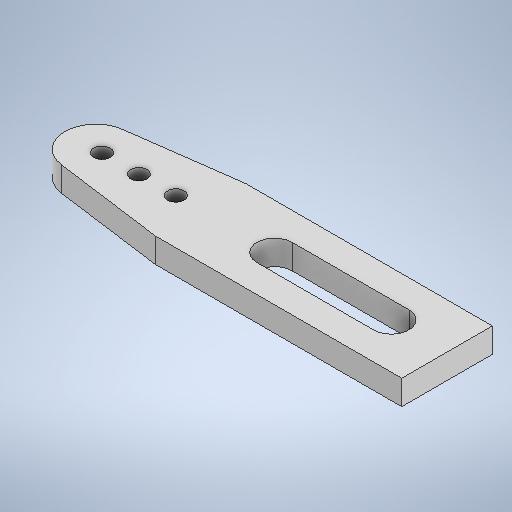
# Autodesk Inventor part: MMAE 232 Assignment 2_Servo Horn 1 - Dylan Tamras
Saved by Autodesk Inventor 2025.2 (Build 292293000, 293)
## iProperties
Created: 2025-01-18
Part Number: MMAE 232 Assignment 2_Servo Horn 1 - Dylan Tamras
Material: Generic
Document SubType Name: Modeling
Designer: Dylan
Density: 1 g/cm^3
Appearance: Default
Author: VRK99-0110
Title: Servo - Horn 1
Autodesk Inventor part; units mm, degrees
ref_plane "YZ Plane" through (0, 0, 0) normal (1, 0, 0) x (0, 1, 0)
ref_plane "XZ Plane" through (0, 0, 0) normal (0, 1, 0) x (-1, 0, 0)
ref_plane "XY Plane" through (0, 0, 0) normal (0, 0, 1) x (1, 0, 0)
sketch "Sketch1" plane through (0, 0, 0) normal (0, 1, 0) x (-1, 0, 0)
  line L0 (0, 0) -> (20, 0)
  line L1 (0, 0) -> (0, -7.35)
  line L2 (0, -7.35) -> (20, -7.35)
  circle A0 centre (28, -3.675) radius 3
  line L3 (20, -7.35) -> (28, -6.675)
  line L4 (20, 0) -> (28, -0.675)
  dimension "d0" = 20
  dimension "d1" = 7.35
  constraints: 10 end point, 2 point on circle, 1 centre point, 1 horizontal, 1 perpendicular, 1 vertical
  measures "d0" distance of L0.start L0.end
  measures "d1" distance of L0.start L1.end
extrude "Extrusion1" add sketch "Sketch1" along normal blind 2
sketch "Sketch3" plane through (0, 2, 0) normal (0, 1, 0) x (1, 0, 0)
  line L0 (0, 0) -> (0, 7.35) projected
  line L1 (-4.5, 2.25) -> (-14, 2.25)
  line L2 (0, 0) -> (0, 3.68)
  line L3 (0, 0) -> (0, 5.1)
  line L4 (-4.5, 5.1) -> (-14, 5.1)
  line L5 (0, 7.35) -> (-20, 7.35) projected
  line L6 (-20, 0) -> (0, 0) projected
  arc A0 (-14, 5.1) -> (-14, 2.25) centre (-14, 3.675) ccw
  arc A1 (-4.5, 2.25) -> (-4.5, 5.1) centre (-4.525, 3.675) ccw
  constraints: 8 end point, 4 point on circle, 2 centre point, 2 point on line, 2 tangent
extrude "Extrusion3" cut sketch "Sketch3" against normal blind 10
sketch "Sketch4" plane through (0, 2, 0) normal (0, 1, 0) x (1, 0, 0)
  line L0 (0, 0) -> (-28, 0)
  line L1 (-20, 0) -> (0, 0) projected
  arc A0 (-28, 6.675) -> (-28, 0.675) centre (-28, 3.675) ccw projected
  line L2 (-28, 0) -> (-28, 6.675)
  dimension "d20" = 28
  constraints: 4 end point, 1 collinear
  measures "d20" distance of L0.start L0.end
extrude "Extrusion4" cut sketch "Sketch4" against normal blind 10
sketch "Sketch5" plane through (0, 2, 0) normal (0, 1, 0) x (1, 0, 0)
  line L0 (-28, 0.675) -> (-20, 0) projected
  line L1 (-20, 0) -> (-20, 7.35)
  line L2 (-20, 7.35) -> (-28, 6.675) projected
  line L3 (-20, 7.35) -> (-28, 6.675)
  line L4 (-28, 6.675) -> (-28, 0.675)
  line L5 (-28, 0.675) -> (-20, 0)
  point P0 (0, 0)
  constraints: 8 end point, 1 collinear, 1 parallel
extrude "Extrusion5" cut sketch "Sketch5" against normal blind 10
sketch "Sketch7" plane through (0, 2, 0) normal (0, 1, 0) x (1, 0, 0)
  line L0 (0, 0) -> (0, 3.675)
  circle A0 centre (-28.5, 3.675) radius 2.5
  line L1 (-20, 0) -> (0, 0) projected
  line L2 (-20, 0) -> (-28.8358, 1.1977)
  line L3 (0, 7.35) -> (-20, 7.35) projected
  line L4 (-20, 7.35) -> (-28.8358, 6.1523)
  line L5 (-20, 7.35) -> (-20, 0) projected
  line L6 (-20, 7.35) -> (-20, 0)
  dimension "d42" = 5
  constraints: 8 end point, 2 point on circle, 2 tangent, 1 centre point, 1 collinear
  measures "d42" diameter of A0
extrude "Extrusion6" add sketch "Sketch7" against normal blind 2
sketch "Sketch8" plane through (0, 2, 0) normal (0, 1, 0) x (1, 0, 0)
  line L0 (0, 0) -> (0, 7.35) projected
  circle A0 centre (-22, 3.675) radius 0.67
  circle A1 centre (-25, 3.675) radius 0.67
  circle A2 centre (-28, 3.675) radius 0.67
  dimension "d46" = 1.34
  dimension "d48" = 1.34
  dimension "d50" = 1.34
  constraints: 3 centre point
  measures "d46" diameter of A0
  measures "d48" diameter of A1
  measures "d50" diameter of A2
extrude "Extrusion7" cut sketch "Sketch8" against normal blind 2
body "Solid1"
